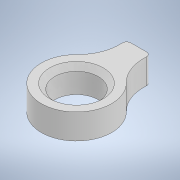
# Autodesk Inventor part: thumbscrew_converter_M3
Saved by Autodesk Inventor 2022 (Build 260153000, 153)
## iProperties
Created: 2020-07-20
Part Number: thumbscrew_converter_M3
Material: Generic
Document SubType Name: Modeling
Designer: Daniel
Density: 1 g/cm^3
Appearance: Default
Author: Daniel
Autodesk Inventor part; units mm, degrees
ref_plane "YZ Plane" through (0, 0, 0) normal (1, 0, 0) x (0, 1, 0)
ref_plane "XZ Plane" through (0, 0, 0) normal (0, 1, 0) x (-1, 0, 0)
ref_plane "XY Plane" through (0, 0, 0) normal (0, 0, 1) x (1, 0, 0)
sketch "Sketch1" plane through (0, 0, 0) normal (0, 1, 0) x (-1, 0, 0)
  circle A0 centre (0, 0) radius 2.6
  circle A1 centre (0, 0) radius 4.2
  line L0 (1.5, -3.923) -> (-1.5, -3.923)
  line L1 (-1.5, -3.923) -> (-1.5, -7.423)
  line L2 (-1.5, -7.423) -> (1.5, -7.423)
  line L3 (1.5, -7.423) -> (1.5, -3.923)
  line L4 (0, 0) -> (0, -7.423)
  arc A2 (2.9348, -3.0045) -> (1.5, -7.423) centre (6.4286, -6.5812) ccw
  arc A3 (-1.5, -7.423) -> (-2.9348, -3.0045) centre (-6.4286, -6.5812) ccw
  point P0 (1.5, -7.423)
  point P1 (-1.5, -5.7395)
  dimension "d0" = 5.2
  dimension "d1" = 1.6
  dimension "d2" = 1.5
  dimension "d3" = 3.5
  dimension "d4" = 5
  dimension "d6" = 5
  constraints: 10 end point, 8 point on circle, 4 centre point, 2 parallel, 2 tangent, 1 coincident, 1 horizontal, 1 horizontal alignment, 1 midpoint, 1 perpendicular, 1 point on line
  measures "d0" diameter of A0
  measures "d1" radial gap between concentric circles of A0 A1
  measures "d2" distance between parallel lines of L4 L3
  measures "d3" distance of L2.end L0.start
  measures "d4" radius of A2
  measures "d6" radius of A3
extrude "Extrusion1" add sketch "Sketch1" along normal blind 3 contours A1 L0 | A1 L1 A3 | A2 L3 A1 | L0 L4 A1 | A1 L4 L2 A3 L1 | L3 A2 L2 L4 A1 | A1 L4 L0
fillet "Fillet2" radius 0.5 2 edges at (1.5, 1.5, -7.423) (-1.5, 1.5, -7.423)
chamfer "Chamfer1" distance 0.6 angle 45 1 edges at (2.6, 3, 0)
equation "\"d0\" = d"
equation "\"d6\" = d4"
equation "\"d7\" = dep"
equation "\"d\" = 5.2"
equation "\"dep\" = 3"
body "Solid1"
